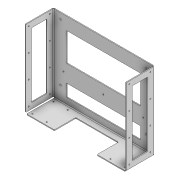
# Autodesk Inventor part: Display_Mount_B
Saved by Autodesk Inventor 2020 (Build 240168000, 168)
## iProperties
Created: 2021-12-05
Part Number: Display_Mount_B
Material: 一般
Document SubType Name: Sheet Metal
Designer: ken113
Density: 1 g/cm^3
Sheet Metal Rule: Default_mm
Appearance: 既定
Author: ken113
Autodesk Inventor part; units mm, degrees
ref_plane "YZ Plane" through (0, 0, 0) normal (1, 0, 0) x (0, 1, 0)
ref_plane "XZ Plane" through (0, 0, 0) normal (0, 1, 0) x (-1, 0, 0)
ref_plane "XY Plane" through (0, 0, 0) normal (0, 0, 1) x (1, 0, 0)
sketch "スケッチ1" plane through (0, 0, 0) normal (0, 0, 1) x (1, 0, 0)
  line L0 (172, -133.5) -> (-172, -133.5)
  line L1 (-172, -133.5) -> (-172, 133.5)
  line L2 (-172, 133.5) -> (172, 133.5)
  line L3 (172, 133.5) -> (172, -133.5)
  line L4 (172, -133.5) -> (-172, 133.5) construction
  line L5 (-172, -133.5) -> (172, 133.5) construction
  point P0 (0, 0)
  dimension "d0" = 267
  dimension "d1" = 344
  measures "d0" distance of L0.end L1.end
  measures "d1" distance of L1.end L2.end
extrude "プレート1" add sketch "スケッチ1" along normal blind 3
sketch "スケッチ2" plane through (172, -136.5, 6) normal (0, -1, 0) x (1, 0, 0)
  line L0 (-344, 0) -> (0, 0)
  line L1 (0, 0) -> (0, 94)
  line L2 (0, 94) -> (-344, 94)
  line L3 (-344, 94) -> (-344, 0)
  constraints: 6 end point, 1 horizontal, 1 perpendicular, 1 vertical
edge flange "フランジ1" height 100 angle 90 thickness 3 bend radius 3 thickness toward (0, -1, 0) relief straight relief width 3 relief depth 1.5 edges at (0, -133.5, 3) wall of the first edge with corners at (-172, -136.5, 6) (172, -136.5, 6) (172, -136.5, 100) (-172, -136.5, 100)
bend "曲げ1"
corner "コーナー1"
sketch "スケッチ3" plane through (0, 0, 3) normal (0, 0, 1) x (1, 0, 0)
  line L0 (150, -86.5) -> (-150, -86.5)
  line L1 (-150, -86.5) -> (-150, 113.5)
  line L2 (-150, 113.5) -> (150, 113.5)
  line L3 (150, 113.5) -> (150, -86.5)
  line L4 (150, -86.5) -> (-150, 113.5) construction
  line L5 (-150, -86.5) -> (150, 113.5) construction
  line L6 (172, -133.5) -> (-172, -133.5) projected
  line L7 (-172, 133.5) -> (172, 133.5) projected
  point P0 (0, 0)
  point P1 (0, 13.5)
  point P2 (0, 13.5)
  dimension "d13" = 300
  dimension "d14" = 200
  dimension "d51" = 120
  constraints: 12 end point, 3 midpoint, 2 parallel, 1 horizontal, 1 perpendicular, 1 vertical alignment
  measures "d13" distance of L0.start L0.end
  measures "d14" distance of L0.end L1.end
  measures "d51" distance from line of L7 point (0, 13.5)
hole "穴1" at (-150, 113.5, 3) at (-150, -86.5, 3) at (150, -86.5, 3) at (150, 113.5, 3) direction (0, 0, -1) diameter 6.2 depth 3 tip angle 118
sketch "スケッチ4" plane through (0, 0, 3) normal (0, 0, 1) x (1, 0, 0)
  line L0 (130, -10.3) -> (-130, -10.3)
  line L1 (-130, -10.3) -> (-130, 89.7)
  line L2 (-130, 89.7) -> (130, 89.7)
  line L3 (130, 89.7) -> (130, -10.3)
  line L4 (130, -10.3) -> (-130, 89.7) construction
  line L5 (-130, -10.3) -> (130, 89.7) construction
  circle A0 centre (-150, 113.5) radius 3.1 projected
  point P0 (0, 0)
  point P1 (0, 39.7)
  point P2 (0, 39.7)
  dimension "d23" = 100
  dimension "d24" = 23.8
  dimension "d25" = 260
  constraints: 12 end point, 3 midpoint, 2 parallel, 1 horizontal, 1 perpendicular, 1 vertical alignment
  measures "d23" distance of L2.end L0.start
  measures "d24" distance from line of L2 A0.centre
  measures "d25" distance of L1.end L2.end
extrude "押し出し1" cut sketch "スケッチ4" against normal through all contours L0 L1 L2 L3
fillet "フィレット1" radius 2 4 edges at (130, -10.3, 1.5) (130, 89.7, 1.5) (-130, 89.7, 1.5) (-130, -10.3, 1.5)
sketch "スケッチ6" plane through (175, 133.5, 6) normal (1, 0, 0) x (0, 1, 0)
  line L0 (-267, 0) -> (0, 0)
  line L1 (0, 0) -> (0, 94)
  line L2 (0, 94) -> (-267, 94)
  line L3 (-267, 94) -> (-267, 0)
  constraints: 6 end point, 1 horizontal, 1 perpendicular, 1 vertical
edge flange "フランジ2" height 100 angle 90 thickness 3 bend radius 3 thickness toward (1, 0, 0) relief straight relief width 3 relief depth 1.5 corner gap 3 corner form 0 edges at (172, 0, 3) (-172, 0, 3) wall of the first edge with corners at (175, -133.5, 6) (175, 133.5, 6) (175, 133.5, 100) (175, -133.5, 100)
bend "曲げ2"
corner "コーナー2"
fillet "フィレット2" radius 2 6 edges at (-176.5, 133.5, 100) (-176.5, -133.5, 100) (-172, -138, 100) (172, -138, 100) (176.5, -133.5, 100) (176.5, 133.5, 100)
sketch "スケッチ7" plane through (-178, -133.5, 6) normal (-1, 0, 0) x (0, 0, 1)
  arc A0 (92, 0) -> (94, 2) centre (92, 2) ccw projected
  line L0 (94, 265) -> (94, 2) projected
  arc A1 (94, 265) -> (92, 267) centre (92, 265) ccw projected
  line L1 (0, 267) -> (92, 267) projected
  line L2 (0, 267) -> (0, 0) projected
  line L3 (92, 0) -> (0, 0) projected
  line L4 (10, 257) -> (84, 257)
  line L5 (84, 257) -> (84, 13)
  line L6 (84, 13) -> (10, 13)
  line L7 (10, 13) -> (10, 257)
  line L8 (10, 94.3333) -> (84, 94.3333)
  line L9 (84, 94.3333) -> (84, 175.6667)
  line L10 (84, 175.6667) -> (10, 175.6667)
  line L11 (10, 175.6667) -> (10, 94.3333)
  point P0 (-6, 133.5)
  dimension "d52" = 10
  dimension "d53" = 10
  dimension "d54" = 10
  dimension "d55" = 13
  dimension "d56" = 244
  dimension "d57" = 81.3333
  dimension "d58" = 81.3333
  constraints: 16 end point, 4 parallel, 2 horizontal, 2 perpendicular, 2 point on line
  measures "d52" distance between parallel lines of L7 L2
  measures "d53" distance between parallel lines of L1 L4
  measures "d54" distance between parallel lines of L0 L5
  measures "d55" distance between parallel lines of L6 L3
  measures "d56" distance of L4.end L5.end
  measures "d57" distance between parallel lines of L4 L10
  measures "d58" distance between parallel lines of L10 L8
hole "穴3" at (-178, -120.5, 16) at (-178, -120.5, 90) at (-178, -39.1667, 90) at (-178, -39.1667, 16) at (-178, 42.1667, 16) at (-178, 42.1667, 90) at (-178, 123.5, 90) at (-178, 123.5, 16) direction (1, 0, 0) diameter 4.134 end through all thread size "M5x0.8" class "6H" standard "ISO Metric profile"
sketch "スケッチ8" plane through (-172, -139.5, 6) normal (0, -1, 0) x (1, 0, 0)
  arc A0 (344, 92) -> (342, 94) centre (342, 92) ccw projected
  line L0 (2, 94) -> (342, 94) projected
  arc A1 (2, 94) -> (0, 92) centre (2, 92) ccw projected
  line L1 (0, 0) -> (0, 92) projected
  line L2 (0, 0) -> (344, 0) projected
  line L3 (344, 92) -> (344, 0) projected
  line L4 (10, 84) -> (60, 84)
  line L5 (60, 84) -> (60, 10)
  line L6 (60, 10) -> (10, 10)
  line L7 (10, 10) -> (10, 84)
  line L8 (284, 10) -> (334, 10)
  line L9 (334, 10) -> (334, 84)
  line L10 (334, 84) -> (284, 84)
  line L11 (284, 84) -> (284, 10)
  point P0 (172, -6)
  dimension "d66" = 50
  dimension "d67" = 50
  dimension "d68" = 10
  dimension "d69" = 10
  dimension "d70" = 10
  dimension "d71" = 10
  constraints: 16 end point, 4 parallel, 2 horizontal, 2 horizontal alignment, 2 perpendicular, 1 point on line
  measures "d66" distance of L4.start L4.end
  measures "d67" distance of L9.end L10.end
  measures "d68" distance between parallel lines of L6 L2
  measures "d69" distance between parallel lines of L0 L10
  measures "d70" distance between parallel lines of L3 L9
  measures "d71" distance between parallel lines of L1 L7
hole "穴4" at (-162, -139.5, 16) at (-112, -139.5, 90) at (-112, -139.5, 16) at (-162, -139.5, 90) at (112, -139.5, 16) at (162, -139.5, 16) at (162, -139.5, 90) at (112, -139.5, 90) direction (0, 1, 0) diameter 4.134 end through all thread size "M5x0.8" class "6H" standard "ISO Metric profile"
sketch "スケッチ9" plane through (-178, -133.5, 6) normal (-1, 0, 0) x (0, 0, 1)
  circle A0 centre (84, 257) radius 2.067 projected
  circle A1 centre (10, 175.6667) radius 2.067 projected
  circle A2 centre (84, 94.3333) radius 2.067 projected
  circle A3 centre (10, 13) radius 2.067 projected
  circle A4 centre (84, 13) radius 2.067 projected
  circle A5 centre (10, 94.3333) radius 2.067 projected
  circle A6 centre (84, 175.6667) radius 2.067 projected
  circle A7 centre (10, 257) radius 2.067 projected
  arc A8 (92, 0) -> (94, 2) centre (92, 2) ccw projected
  line L0 (94, 265) -> (94, 2) projected
  arc A9 (94, 265) -> (92, 267) centre (92, 265) ccw projected
  line L1 (0, 267) -> (92, 267) projected
  line L2 (0, 267) -> (0, 0) projected
  line L3 (92, 0) -> (0, 0) projected
  line L4 (20, 247) -> (74, 247)
  line L5 (74, 247) -> (74, 20)
  line L6 (74, 20) -> (20, 20)
  line L7 (20, 20) -> (20, 247)
  point P0 (-6, 133.5)
  dimension "d79" = 20
  dimension "d80" = 20
  dimension "d81" = 20
  dimension "d82" = 20
  constraints: 8 end point, 2 parallel, 1 horizontal, 1 perpendicular
  measures "d79" distance between parallel lines of L0 L5
  measures "d80" distance between parallel lines of L2 L7
  measures "d81" distance between parallel lines of L1 L4
  measures "d82" distance between parallel lines of L3 L6
extrude "押し出し2" cut sketch "スケッチ9" against normal through all contours L4 L5 L6 L7
fillet "フィレット3" radius 2 8 edges at (-176.5, 113.5, 26) (-176.5, 113.5, 80) (-176.5, -113.5, 26) (-176.5, -113.5, 80) (176.5, -113.5, 26) (176.5, -113.5, 80) (176.5, 113.5, 80) (176.5, 113.5, 26)
sketch "スケッチ11" plane through (0, 0, 3) normal (0, 0, 1) x (1, 0, 0)
  line L0 (130, 87.7) -> (130, -8.3) projected
  arc A0 (128, -10.3) -> (130, -8.3) centre (128, -8.3) ccw projected
  line L1 (128, -10.3) -> (-128, -10.3) projected
  arc A1 (-130, -8.3) -> (-128, -10.3) centre (-128, -8.3) ccw projected
  line L2 (-130, -8.3) -> (-130, 87.7) projected
  arc A2 (-128, 89.7) -> (-130, 87.7) centre (-128, 87.7) ccw projected
  line L3 (-128, 89.7) -> (128, 89.7) projected
  arc A3 (130, 87.7) -> (128, 89.7) centre (128, 87.7) ccw projected
  circle A4 centre (150, -86.5) radius 3.1 projected
  circle A5 centre (-150, 113.5) radius 3.1 projected
  circle A6 centre (-150, -86.5) radius 3.1 projected
  circle A7 centre (150, 113.5) radius 3.1 projected
  line L4 (-172, -133.5) -> (-172, 133.5) projected
  line L5 (172, -133.5) -> (-172, -133.5) projected
  line L6 (172, 133.5) -> (172, -133.5) projected
  line L7 (-172, 133.5) -> (172, 133.5) projected
  point P0 (0, 0)
  point P1 (-140, -40.3)
  point P2 (0, -40.3)
  point P3 (140, -40.3)
  dimension "d89" = 140
  dimension "d94" = 30
  constraints: 1 horizontal, 1 vertical alignment, 2 other
  measures "d89" distance of point (-140, -40.3) point (0, -40.3)
  measures "d94" distance from line of L1 point (-140, -40.3)
hole "穴5" at (-140, -40.3, 3) at (0, -40.3, 3) at (140, -40.3, 3) direction (0, 0, -1) diameter 4.3 end through all
sketch "スケッチ12" plane through (0, 0, 0) normal (0, 0, -1) x (-1, 0, 0)
  circle A0 centre (0, -40.3) radius 2.15 projected
  circle A1 centre (140, -40.3) radius 2.15 projected
  circle A2 centre (-140, -40.3) radius 2.15 projected
  line L0 (-130, -8.3) -> (-130, 87.7) projected
  arc A3 (-128, 89.7) -> (-130, 87.7) centre (-128, 87.7) ccw projected
  line L1 (-128, 89.7) -> (128, 89.7) projected
  arc A4 (130, 87.7) -> (128, 89.7) centre (128, 87.7) ccw projected
  line L2 (130, 87.7) -> (130, -8.3) projected
  arc A5 (128, -10.3) -> (130, -8.3) centre (128, -8.3) ccw projected
  line L3 (128, -10.3) -> (-128, -10.3) projected
  arc A6 (-130, -8.3) -> (-128, -10.3) centre (-128, -8.3) ccw projected
  circle A7 centre (-150, -86.5) radius 3.1 projected
  circle A8 centre (150, 113.5) radius 3.1 projected
  circle A9 centre (150, -86.5) radius 3.1 projected
  circle A10 centre (-150, 113.5) radius 3.1 projected
  line L4 (-172, -133.5) -> (172, -133.5) projected
  line L5 (172, -133.5) -> (172, 133.5) projected
  line L6 (172, 133.5) -> (-172, 133.5) projected
  line L7 (-172, 133.5) -> (-172, -133.5) projected
  point P0 (0, 0)
hole "穴6" at (140, -40.3, 0) at (0, -40.3, 0) at (-140, -40.3, 0) direction (0, 0, 1) diameter 4.2 end through all countersink diameter 8 countersink angle 90
sketch "スケッチ13" plane through (0, 0, 3) normal (0, 0, 1) x (1, 0, 0)
  line L0 (-130, -113.5) -> (130, -113.5)
  line L1 (130, -113.5) -> (130, -70.3)
  line L2 (130, -70.3) -> (-130, -70.3)
  line L3 (-130, -70.3) -> (-130, -113.5)
  circle A0 centre (0, -40.3) radius 2.15 projected
  line L4 (172, -133.5) -> (-172, -133.5) projected
  point P0 (0, 0)
  point P1 (-130, 87.7)
  point P2 (130, -8.3)
  dimension "d109" = 30
  dimension "d110" = 20
  constraints: 8 end point, 2 parallel, 2 vertical alignment, 1 horizontal, 1 perpendicular
  measures "d109" distance from line of A0.centre L2
  measures "d110" distance between parallel lines of L0 L4
extrude "押し出し3" cut sketch "スケッチ13" against normal blind 10 contours L3 L2 L1 L0
fillet "フィレット4" radius 2 4 edges at (-130, -70.3, 1.5) (-130, -113.5, 1.5) (130, -113.5, 1.5) (130, -70.3, 1.5)
sketch "スケッチ14" plane through (-172, -136.5, 6) normal (0, 1, 0) x (1, 0, 0)
  line L0 (2, -94) -> (342, -94) projected
  line L1 (97, -94) -> (247, -94)
  line L2 (247, -94) -> (247, -19)
  line L3 (247, -19) -> (97, -19)
  line L4 (97, -19) -> (97, -94)
  line L5 (0, 3) -> (344, 3) projected
  point P0 (172, 6)
  point P1 (172, 6)
  dimension "d114" = 150
  dimension "d115" = 75
  dimension "d116" = 22
  constraints: 8 end point, 2 parallel, 1 coincident, 1 horizontal, 1 perpendicular, 1 point on line
  measures "d114" distance between parallel lines of L2 L4
  measures "d115" distance from line of L2 point (172, 6)
  measures "d116" distance between parallel lines of L3 L5
extrude "押し出し4" cut sketch "スケッチ14" against normal blind 10
fillet "フィレット5" radius 2 4 edges at (-75, -138, 100) (-75, -138, 25) (75, -138, 100) (75, -138, 25)
equation "\"d21\" = Thickness"
equation "\"d57\" = 0.333333 * d56"
equation "\"d58\" = d57"
equation "\"d2\" = Thickness"
equation "\"d3\" = BendReliefWidth"
equation "\"d4\" = BendReliefDepth"
equation "\"d5\" = MinimumRemnant"
equation "\"d6\" = TransitionRadius"
equation "\"d9\" = BendRadius"
equation "\"d10\" = CornerReliefSize"
equation "\"d11\" = GapSize"
equation "\"d12\" = JacobiRadiusSize"
equation "\"d40\" = BendReliefWidth"
equation "\"d41\" = BendReliefDepth"
equation "\"d42\" = MinimumRemnant"
equation "\"d43\" = TransitionRadius"
equation "\"d46\" = BendRadius"
equation "\"d47\" = CornerReliefSize"
equation "\"d48\" = GapSize"
equation "\"d49\" = JacobiRadiusSize"
equation "\"BendRadius\" = Thickness"
equation "\"BendReliefWidth\" = Thickness"
equation "\"BendReliefDepth\" = 0.5 * Thickness"
equation "\"CornerReliefSize\" = 4 * Thickness"
equation "\"MinimumRemnant\" = 2 * Thickness"
equation "\"TransitionRadius\" = BendRadius"
equation "\"JacobiRadiusSize\" = BendRadius"
equation "\"GapSize\" = Thickness"
equation "\"Thickness\" = 3"
